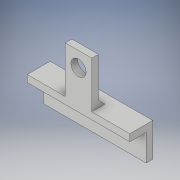
# Autodesk Inventor part: NewNewMechanism
Saved by Autodesk Inventor 2017 (Build 210142000, 142)
## iProperties
Created: 2020-02-07
Part Number: NewNewMechanism
Material: Generic
Document SubType Name: Modeling
Designer: S347110131
Density: 1 g/cm^3
Appearance: Default
Author: S347110131
Autodesk Inventor part; units mm, degrees
ref_plane "YZ Plane" through (0, 0, 0) normal (1, 0, 0) x (0, 1, 0)
ref_plane "XZ Plane" through (0, 0, 0) normal (0, 1, 0) x (-1, 0, 0)
ref_plane "XY Plane" through (0, 0, 0) normal (0, 0, 1) x (1, 0, 0)
sketch "Sketch2" plane through (0, 0, 0) normal (0, 0, 1) x (1, 0, 0)
  circle A0 centre (0, 0) radius 406.4
  line L0 (-704.85, -381) -> (704.85, -381)
  line L1 (704.85, -381) -> (704.85, 381)
  line L2 (-704.85, 381) -> (-704.85, -381)
  line L3 (-704.85, -381) -> (704.85, 381) construction
  line L4 (704.85, -381) -> (-704.85, 381) construction
  line L5 (0, 381) -> (-98.1878, 381)
  line L6 (0, 394.3604) -> (-98.1878, 394.3604)
  line L7 (-98.1878, 394.3604) -> (-98.1878, 381)
  line L8 (0, 394.3604) -> (98.1878, 394.3604)
  line L9 (98.1878, 394.3604) -> (98.1878, 381)
  line L10 (-98.1878, 381) -> (98.1878, 381)
  line L11 (-98.1878, 381) -> (98.1878, 381)
  line L12 (-98.1878, 394.3604) -> (98.1878, 394.3604)
  line L13 (98.1878, 394.3604) -> (98.1878, 381)
  line L14 (-98.1878, 394.3604) -> (-98.1878, 381)
  line L15 (-141.4212, 381) -> (-704.85, 381)
  line L16 (704.85, 381) -> (141.4212, 381)
  line L17 (98.1878, 381) -> (-98.1878, 381)
  dimension "d0" = 812.8
  dimension "d1" = 1409.7
  dimension "d2" = 762
  dimension "d9" = 394.3604
  constraints: 36 end point, 8 collinear, 7 perpendicular, 4 parallel, 4 point on circle, 3 midpoint, 2 horizontal, 1 centre point, 1 coincident
  measures "d0" diameter of A0
  measures "d1" distance of L2.start L1.end
  measures "d2" distance of L1.end L0.end
  measures "d9" distance of A0.centre L6.start
extrude "Extrusion1" add sketch "Sketch2" along normal blind 31.242 contours L9 L10 L5 L7 L6 L8
sketch "Sketch4" plane through (0, 0, 31.242) normal (0, 0, 1) x (1, 0, 0)
  circle A0 centre (0, 0) radius 406.4
  line L0 (98.1878, 394.3604) -> (-98.1878, 394.3604) projected
  circle A1 centre (0, 454.5584) radius 14.5542
  line L1 (25.4, 394.3604) -> (-25.4, 394.3604)
  line L2 (-25.4, 394.3604) -> (-25.4, 483.2604)
  line L3 (-25.4, 483.2604) -> (25.4, 483.2604)
  line L4 (25.4, 483.2604) -> (25.4, 394.3604)
  line L5 (0, 0) -> (0, 517.5127)
  arc A2 (25.4, 410.5643) -> (-25.4, 410.5643) centre (0, 454.5584) ccw
  line L6 (-98.1878, 381) -> (98.1878, 381) projected
  dimension "d10" = 812.8
  dimension "d12" = 60.198
  dimension "d13" = 29.1084
  dimension "d14" = 50.8
  dimension "d15" = 88.9
  dimension "d16" = 25.4
  dimension "d27" = 13.3604
  dimension "d28" = 50.8
  constraints: 10 end point, 3 centre point, 3 point on line, 2 coincident, 2 parallel, 2 point on circle, 1 horizontal, 1 perpendicular, 1 vertical
  measures "d10" diameter of A0
  measures "d12" distance from line of A2.centre L0
  measures "d13" diameter of A1
  measures "d14" distance of L2.end L3.end
  measures "d15" distance of L1.end L2.end
  measures "d16" distance between parallel lines of L5 L4
  measures "d27" distance between parallel lines of L6 L0
  measures "d28" radius of A2
extrude "Extrusion2" add sketch "Sketch4" against normal blind 12.7 contours L4 L0 L5 A0 | A0 L5 A1 L3 L4 | L2 L3 L5 A1 A0 | A0 L5 L0 L2
sketch "Sketch7" plane through (0, 0, 0) normal (0, 0, -1) x (-1, 0, 0)
  line L0 (98.1878, 394.3604) -> (98.1878, 381) projected
  line L1 (98.1878, 394.3604) -> (-98.1878, 394.3604)
  line L2 (-98.1878, 394.3604) -> (-98.1878, 330.2)
  line L3 (-98.1878, 330.2) -> (98.1878, 330.2)
  line L4 (98.1878, 330.2) -> (98.1878, 394.3604)
  line L5 (98.1878, 381) -> (-98.1878, 381) projected
  point P0 (0, 0)
  dimension "d23" = 50.8
  dimension "d24" = 64.1604
  constraints: 8 end point, 2 parallel, 1 horizontal, 1 perpendicular
  measures "d23" distance between parallel lines of L5 L3
  measures "d24" distance between parallel lines of L3 L1
extrude "Extrusion5" add sketch "Sketch7" along normal blind 12.7
sketch "Sketch8" plane through (0, 0, -12.7) normal (0, 0, -1) x (-1, 0, 0)
  line L0 (98.1878, 394.3604) -> (-98.1878, 394.3604) projected
  circle A0 centre (0, 362.2802) radius 3.175
  point P0 (0, 0)
  dimension "d31" = 6.35
  constraints: 1 centre point
  measures "d31" diameter of A0
extrude "Extrusion6" cut sketch "Sketch8" against normal blind 12.7
thread "Thread1" size "1/4-20 UNC" class "2B" standard "ANSI Unified Screw Threads" full length
sketch "Sketch9" plane through (-25.4, 394.3604, 31.242) normal (-1, 0, 0) x (0, 0, 1)
  line L0 (0, 88.9) -> (-12.7, 88.9) projected
  line L1 (-12.7, 88.9) -> (-12.7, 0) projected
  line L2 (-12.7, 12.7) -> (-12.7, 0)
  line L3 (-12.7, 0) -> (-25.4, 0)
  line L4 (-43.942, 0) -> (0, 0) projected
  line L5 (-25.4, 0) -> (-12.7, 12.7)
  point P0 (-31.242, -394.3604)
  dimension "d36" = 12.7
  dimension "d37" = 45
  constraints: 6 end point, 1 point on line, 1 vertical
  measures "d36" distance of L1.end L3.end
  measures "d37" angle of L3 L5
extrude "Extrusion7" add sketch "Sketch9" against normal blind 2.54
sketch "Sketch10" plane through (25.4, 394.3604, 31.242) normal (1, 0, 0) x (0, 0, -1)
  line L0 (25.4, 0) -> (12.7, 0) projected
  line L1 (25.4, 0) -> (12.7, 12.7) projected
  line L2 (12.7, 0) -> (12.7, 12.7)
  line L3 (12.7, 12.7) -> (25.4, 0)
  line L4 (25.4, 0) -> (12.7, 0)
  point P0 (31.242, -394.3604)
  constraints: 6 end point, 1 collinear, 1 perpendicular, 1 vertical
extrude "Extrusion8" add sketch "Sketch10" against normal blind 2.54
body "Solid1"
